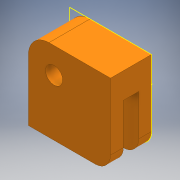
# Autodesk Inventor part: Plate Adapter 5.0
Saved by Autodesk Inventor 2017 (Build 210142000, 142)
## iProperties
Created: 2017-04-29
Part Number: Plate Adapter 5.0
Material: Generic
Document SubType Name: Modeling
Designer: gilef
Density: 1 g/cm^3
Appearance: Orange
Author: gilef
Autodesk Inventor part; units mm, degrees
ref_plane "YZ Plane" through (0, 0, 0) normal (1, 0, 0) x (0, 1, 0)
ref_plane "XZ Plane" through (0, 0, 0) normal (0, 1, 0) x (-1, 0, 0)
ref_plane "XY Plane" through (0, 0, 0) normal (0, 0, 1) x (1, 0, 0)
sketch "Sketch1" plane through (0, 0, 0) normal (0, 1, 0) x (-1, 0, 0)
  line L0 (0, 0) -> (8, 0)
  line L1 (0, 0) -> (0, 5)
  line L2 (0, 5) -> (16, 5)
  arc A0 (11, -3) -> (8, 0) centre (8, -3) ccw
  line L3 (11, -3) -> (11, -11)
  line L4 (11, -11) -> (16, -11)
  line L5 (16, -11) -> (16, 5)
  line L6 (0, 0) -> (11, -11)
  dimension "d0" = 5
  dimension "d1" = 5
  dimension "d2" = 8
  dimension "d3" = 3
  dimension "d4" = 8
  constraints: 14 end point, 3 perpendicular, 3 vertical, 2 point on circle, 2 tangent, 1 centre point, 1 horizontal
  measures "d0" distance of L0.start L1.end
  measures "d1" distance of L3.end L4.end
  measures "d2" distance of L0.start L0.end
  measures "d3" radius of A0
  measures "d4" distance of L3.start L3.end
extrude "Extrusion1" add sketch "Sketch1" along normal blind 8 contours L1 L2 L5 L4 L3 A0 L0
sketch "Sketch2" plane through (0, 0, 0) normal (0, -1, 0) x (1, 0, 0)
  line L0 (0, 0) -> (-8, 0) projected
  arc A0 (-8, 0) -> (-11, -3) centre (-8, -3) ccw projected
  line L1 (-11, -3) -> (-11, -11) projected
  line L2 (0, 0) -> (-11, -11)
  line L3 (-11, -11) -> (-11, -3)
  line L4 (-8, 0) -> (0, 0)
  arc A1 (-8, 0) -> (-11, -3) centre (-8, -3) ccw
  line L5 (0, 0) -> (0, -8)
  arc A2 (-3, -11) -> (0, -8) centre (-3, -8) ccw
  line L6 (-3, -11) -> (-11, -11)
  constraints: 10 end point, 4 point on circle, 3 symmetric about line, 2 centre point, 1 coincident, 1 collinear, 1 concentric, 1 perpendicular, 1 point on line, 1 other
extrude "Extrusion2" add sketch "Sketch2" against normal blind 2.5
ref_plane "Work Plane1" through (0, 5.5, 0) normal (0, 1, 0) x (1, 0, 0)
sketch "Sketch3" plane through (0, 5.5, 0) normal (0, 1, 0) x (1, 0, 0)
  line L0 (0, 0) -> (0, 8) projected
  arc A0 (0, 8) -> (-3, 11) centre (-3, 8) ccw projected
  line L1 (-3, 11) -> (-11, 11) projected
  line L2 (-11, 3) -> (-11, 11) projected
  arc A1 (-11, 3) -> (-8, 0) centre (-8, 3) ccw projected
  line L3 (0, 0) -> (-8, 0) projected
extrude "Extrusion3" add sketch "Sketch3" along normal blind 2.5
sketch "Sketch4" plane through (0, 8, 0) normal (0, 1, 0) x (1, 0, 0)
  arc A0 (0, 8) -> (-3, 11) centre (-3, 8) ccw projected
  line L0 (0, -5) -> (0, 8) projected
  line L1 (-3, 11) -> (-16, 11) projected
  line L2 (-16, 11) -> (-16, -5) projected
  line L3 (-16, -5) -> (0, -5) projected
  point P0 (0, 0)
sketch "Sketch5" plane through (0, 8, 0) normal (0, 1, 0) x (1, 0, 0)
  circle A0 centre (-11, 0) radius 1.6667
  line L0 (-16, -5) -> (0, -5) projected
  line L1 (-16, 11) -> (-16, -5) projected
  point P0 (0, 0)
  point P1 (-8, -5)
  point P2 (-16, 3)
  dimension "d21" = 3.3333
  dimension "d22" = 3.3333
  dimension "d23" = 3.3333
  constraints: 1 centre point
  measures "d21" diameter of A0
  measures "d22" distance edge to line of A0 L1
  measures "d23" distance edge to line of A0 L0
extrude "Extrusion4" cut sketch "Sketch5" against normal through all
fillet "Fillet2" radius 0.25 1 edges at (-12.6667, 8, 0)
fillet "Fillet3" radius 4 1 edges at (-16, 4, 5)
equation "\"d1\" = d0"
equation "\"d23\" = d22"
body "Solid1"
